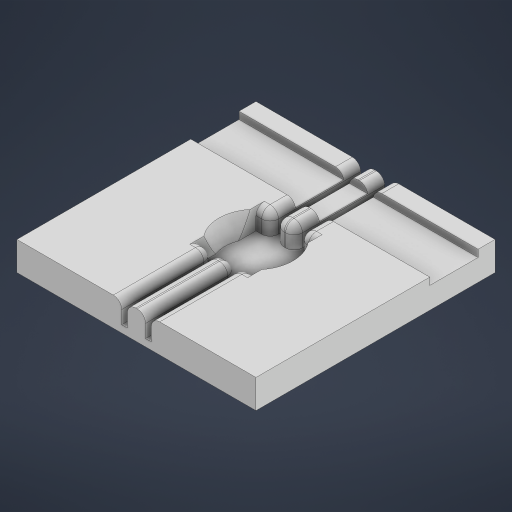
# Autodesk Inventor part: Richtfest
Saved by Autodesk Inventor 2023 (Build 270158030, 158C)
## iProperties
Created: 2022-06-02
Part Number: Richtfest
Material: Generic
Document SubType Name: Modeling
Designer: Simon
Density: 1 g/cm^3
Appearance: Default
Author: Simon
Autodesk Inventor part; units mm, degrees
ref_plane "YZ Plane" through (0, 0, 0) normal (1, 0, 0) x (0, 1, 0)
ref_plane "XZ Plane" through (0, 0, 0) normal (0, 1, 0) x (-1, 0, 0)
ref_plane "XY Plane" through (0, 0, 0) normal (0, 0, 1) x (1, 0, 0)
sketch "Sketch1" plane through (0, 0, 0) normal (0, 1, 0) x (-1, 0, 0)
  line L0 (6.05, 6.05) -> (-6.05, 6.05)
  line L1 (-6.05, 6.05) -> (-6.05, -6.05)
  line L2 (-6.05, -6.05) -> (6.05, -6.05)
  line L3 (6.05, -6.05) -> (6.05, 6.05)
  line L4 (6.05, 6.05) -> (-6.05, -6.05) construction
  line L5 (-6.05, 6.05) -> (6.05, -6.05) construction
  line L6 (25, 25) -> (-25, 25)
  line L7 (-25, 25) -> (-25, -25)
  line L8 (-25, -25) -> (25, -25)
  line L9 (25, -25) -> (25, 25)
  line L10 (25, 25) -> (-25, -25) construction
  line L11 (-25, 25) -> (25, -25) construction
  point P0 (0, 0)
  dimension "d0" = 12.1
  dimension "d1" = 12.1
  dimension "d2" = 50
  dimension "d3" = 50
  constraints: 24 end point, 4 midpoint, 4 parallel, 2 horizontal, 2 perpendicular
  measures "d0" distance of L2.end L1.end
  measures "d1" distance of L1.end L0.end
  measures "d2" distance of L8.end L7.end
  measures "d3" distance of L7.end L6.end
extrude "Extrusion1" add sketch "Sketch1" along normal blind 4.5
sketch "Sketch2" plane through (0, 4.5, 0) normal (0, 1, 0) x (1, 0, 0)
  line L0 (25, 25) -> (-25, 25) projected
  line L1 (-3.1, -25) -> (3.1, -25)
  line L2 (3.1, -25) -> (3.1, 25)
  line L3 (3.1, 25) -> (-3.1, 25)
  line L4 (-3.1, 25) -> (-3.1, -25)
  line L5 (-3.1, -25) -> (3.1, 25) construction
  line L6 (3.1, -25) -> (-3.1, 25) construction
  line L7 (1.9, -25) -> (-1.9, -25)
  line L8 (-1.9, -25) -> (-1.9, 25)
  line L9 (-1.9, 25) -> (1.9, 25)
  line L10 (1.9, 25) -> (1.9, -25)
  line L11 (1.9, -25) -> (-1.9, 25) construction
  line L12 (-1.9, -25) -> (1.9, 25) construction
  point P0 (0, 0)
  dimension "d6" = 6.2
  dimension "d7" = 3.8
  constraints: 24 end point, 4 midpoint, 4 parallel, 2 horizontal, 2 perpendicular, 2 point on line
  measures "d6" distance of L3.end L2.end
  measures "d7" distance of L8.end L9.end
extrude "Extrusion2" cut sketch "Sketch2" against normal blind 4.5 contours L2 L1 L10 L0 | L8 L1 L4 L0
sketch "Sketch3" plane through (0, 0, 0) normal (0, -1, 0) x (1, 0, 0)
  line L0 (-25, -25) -> (-25, 25) projected
  line L1 (25, 25) -> (25, -25) projected
  line L2 (-25, 25) -> (25, 25)
  line L3 (25, 25) -> (25, -25)
  line L4 (25, -25) -> (-25, -25)
  line L5 (-25, -25) -> (-25, 25)
  point P0 (0, 0)
  constraints: 8 end point, 2 parallel, 1 horizontal, 1 perpendicular
extrude "Extrusion3" add sketch "Sketch3" along normal blind 1.5
fillet "Fillet1" radius 1.75 8 edges at (3.1, 4.5, 15.525) (1.9, 4.5, 15.525) (-1.9, 4.5, 15.525) (-3.1, 4.5, 15.525) (3.1, 4.5, -15.525) (1.9, 4.5, -15.525) (-1.9, 4.5, -15.525) (-3.1, 4.5, -15.525)
fillet "Fillet2" radius 1.75 22 edges at (0, 4.5, 6.05) (-1.3874, 3.9874, 6.05) (-1.9, 1.375, 6.05) (1.9, 1.375, 6.05) (1.3874, 3.9874, 6.05) (3.6126, 3.9874, 6.05) (3.1, 1.375, 6.05) (5.45, 4.5, 6.05) (-5.45, 4.5, 6.05) (-3.1, 1.375, 6.05) (-3.6126, 3.9874, 6.05) (5.45, 4.5, -6.05) (3.1, 1.375, -6.05) (3.6126, 3.9874, -6.05) (0, 4.5, -6.05) (1.3874, 3.9874, -6.05) (1.9, 1.375, -6.05) (-1.9, 1.375, -6.05) (-1.3874, 3.9874, -6.05) (-3.6126, 3.9874, -6.05) (-3.1, 1.375, -6.05) (-5.45, 4.5, -6.05)
sketch "Sketch5" plane through (0, 4.5, 0) normal (0, 1, 0) x (1, 0, 0)
  circle A0 centre (0, 0) radius 6.5
  line L0 (4.0811, 5.0591) -> (-4.0811, 5.0591)
  line L1 (4.0811, -5.0591) -> (-4.0811, -5.0591)
  dimension "d17" = 13
  constraints: 4 end point, 4 point on circle, 1 centre point, 1 coincident, 1 horizontal, 1 parallel
  measures "d17" diameter of A0
extrude "Extrusion5" cut sketch "Sketch5" against normal blind 4.5 contours A0 L1 L0
chamfer "Chamfer1" distance 1.25 angle 74.47 1 edges at (6.5, 4.5, 0) measured on face at (7, 4.5, 0)
chamfer "Chamfer2" distance 1.25 angle 74.47 1 edges at (-6.5, 4.5, 0) measured on face at (-7, 4.5, 0)
sketch "Sketch6" plane through (0, 4.5, 0) normal (0, 1, 0) x (1, 0, 0)
  line L0 (-25, -25) -> (-25, 25) projected
  line L1 (24.7, 21.45) -> (-25, 21.45)
  line L2 (-25, 21.45) -> (-25, 11.35)
  line L3 (-25, 11.35) -> (24.7, 11.35)
  line L4 (24.7, 11.35) -> (24.7, 21.45)
  line L5 (-0.15, 7.8) -> (-0.15, 25) projected
  line L6 (24.7, 21.45) -> (-25, 11.35) construction
  line L7 (-25, 21.45) -> (24.7, 11.35) construction
  point P0 (0, 0)
  point P1 (-0.15, 16.4)
  dimension "d26" = 10.1
  constraints: 12 end point, 3 midpoint, 2 parallel, 1 horizontal, 1 perpendicular, 1 point on line
  measures "d26" distance of L2.end L1.end
extrude "Extrusion6" cut sketch "Sketch6" against normal blind 1.5
delete faces "Delete Face1" heal yes whole lump no faces at (24.7, 4, -14.7167)
body "Solid1"
